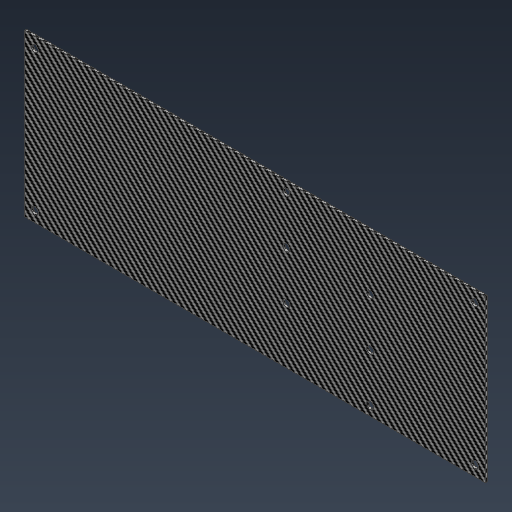
# Autodesk Inventor part: plate3
Saved by Autodesk Inventor 2021 (Build 250183000, 183)
## iProperties
Created: 2021-07-22
Part Number: plate3
Material: CFRP
Document SubType Name: Sheet Metal
Designer: yuta0
Density: 1.43 g/cm^3
Sheet Metal Rule: Default
Appearance: カーボンファイバー
購入先: カーボン
在庫数: 0.0
Author: yuta0
Autodesk Inventor part; units mm, degrees
ref_plane "YZ Plane" through (0, 0, 0) normal (1, 0, 0) x (0, 1, 0)
ref_plane "XZ Plane" through (0, 0, 0) normal (0, 1, 0) x (-1, 0, 0)
ref_plane "XY Plane" through (0, 0, 0) normal (0, 0, 1) x (1, 0, 0)
sketch "スケッチ1" plane through (0, 0, 0) normal (0, 0, 1) x (1, 0, 0)
  line L0 (-110, -38.5) -> (110, -38.5)
  line L1 (110, -38.5) -> (110, 38.5)
  line L2 (110, 38.5) -> (-110, 38.5)
  line L3 (-110, 38.5) -> (-110, -38.5)
  line L4 (-110, -38.5) -> (110, 38.5) construction
  line L5 (110, -38.5) -> (-110, 38.5) construction
  point P0 (0, 0)
  dimension "d0" = 220
  dimension "d1" = 77
  measures "d0" distance of L2.end L1.end
  measures "d1" distance of L1.end L0.end
extrude "プレート1" add sketch "スケッチ1" along normal blind 1
sketch "スケッチ2" plane through (0, 0, 1) normal (0, 0, 1) x (1, 0, 0)
  line L0 (-110, -38.5) -> (-110, 38.5) projected
  line L1 (110, -38.5) -> (-110, -38.5) projected
  line L2 (110, 38.5) -> (110, -38.5) projected
  line L3 (-110, 38.5) -> (110, 38.5) projected
  line L4 (105, 33.5) -> (105, -33.5)
  line L5 (105, -33.5) -> (-105, -33.5)
  line L6 (-105, -33.5) -> (-105, 33.5)
  line L7 (-105, 33.5) -> (105, 33.5)
  point P0 (0, 0)
  dimension "d3" = 5
  constraints: 8 end point, 3 other
  measures "d3" distance between parallel lines of L3 L7
hole "穴1" at (-105, 33.5, 1) at (-105, -33.5, 1) at (105, -33.5, 1) at (105, 33.5, 1) direction (0, 0, -1) diameter 3.4 depth 1 clearance for "Flat Head Machine Screw" size "M3" standard "Ansi Metric M Profile"
sketch "スケッチ3" plane through (0, 0, 1) normal (0, 0, 1) x (1, 0, 0)
  line L0 (55, -34.125) -> (15, -34.125)
  line L1 (15, -34.125) -> (15, -11.875)
  line L2 (15, -11.875) -> (55, -11.875)
  line L3 (55, -11.875) -> (55, -34.125)
  line L4 (55, -34.125) -> (15, -11.875) construction
  line L5 (15, -34.125) -> (55, -11.875) construction
  line L6 (15, 11.125) -> (55, 11.125)
  line L7 (55, 11.125) -> (55, -11.125)
  line L8 (55, -11.125) -> (15, -11.125)
  line L9 (15, -11.125) -> (15, 11.125)
  line L10 (15, 11.125) -> (55, -11.125) construction
  line L11 (55, 11.125) -> (15, -11.125) construction
  line L12 (15, 11.875) -> (55, 11.875)
  line L13 (55, 11.875) -> (55, 34.125)
  line L14 (55, 34.125) -> (15, 34.125)
  line L15 (15, 34.125) -> (15, 11.875)
  line L16 (15, 11.875) -> (55, 34.125) construction
  line L17 (55, 11.875) -> (15, 34.125) construction
  point P0 (0, 0)
  point P1 (35, -23)
  point P2 (35, 0)
  point P3 (35, 0)
  point P4 (35, 23)
  point P5 (35, 23)
  point P6 (35, 0)
  point P7 (35, -23)
  dimension "d11" = 22.25
  dimension "d12" = 40
  dimension "d13" = 40
  dimension "d14" = 22.25
  dimension "d15" = 40
  dimension "d16" = 22.25
  dimension "d17" = 23
  dimension "d18" = 23
  dimension "d20" = 35
  constraints: 36 end point, 10 midpoint, 6 parallel, 3 horizontal, 3 perpendicular, 2 vertical alignment, 1 horizontal alignment
  measures "d11" distance of L0.end L1.end
  measures "d12" distance of L0.start L0.end
  measures "d13" distance of L7.end L8.end
  measures "d14" distance of L6.end L7.end
  measures "d15" distance of L14.end L13.end
  measures "d16" distance of L13.end L12.end
  measures "d17" distance of point (35, 0) point (35, 23)
  measures "d18" distance of point (35, 0) point (35, -23)
  measures "d20" horizontal distance of point (0, 0) point (35, 23)
hole "穴2" at (15, 34.125, 1) at (55, 11.875, 1) at (15, 11.125, 1) at (55, -11.125, 1) at (15, -11.875, 1) at (55, -34.125, 1) direction (0, 0, -1) diameter 3.4 end through all clearance for "Flat Head Machine Screw" size "M3" standard "Ansi Metric M Profile"
equation "\"d9\" = Thickness"
equation "\"d26\" = Thickness"
equation "\"d2\" = Thickness"
equation "\"BendRadius\" = Thickness"
equation "\"BendReliefWidth\" = Thickness"
equation "\"BendReliefDepth\" = 0.5 * Thickness"
equation "\"CornerReliefSize\" = 4 * Thickness"
equation "\"MinimumRemnant\" = 2 * Thickness"
equation "\"TransitionRadius\" = BendRadius"
equation "\"JacobiRadiusSize\" = Thickness"
equation "\"GapSize\" = Thickness"
equation "\"Thickness\" = 1"
